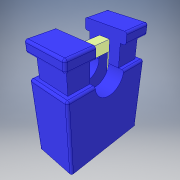
# Autodesk Inventor part: Jumper
Saved by Autodesk Inventor 2018 (Build 220112000, 112)
## iProperties
Created: 2021-02-06
Part Number: Jumper
Material: Všeobecné
Document SubType Name: Modeling
Designer: Jozko Mrkvicka
Density: 1 g/cm^3
Appearance: Výchozí
Author: Jozko Mrkvicka
Autodesk Inventor part; units mm, degrees
ref_plane "YZ Plane" through (0, 0, 0) normal (1, 0, 0) x (0, 1, 0)
ref_plane "XZ Plane" through (0, 0, 0) normal (0, 1, 0) x (-1, 0, 0)
ref_plane "XY Plane" through (0, 0, 0) normal (0, 0, 1) x (1, 0, 0)
sketch "Náčrt1" plane through (0, 0, 0) normal (0, 1, 0) x (-1, 0, 0)
  line L0 (0, 0) -> (2.54, 0)
  line L1 (2.54, 0) -> (2.54, -5.08)
  line L2 (2.54, -5.08) -> (0, -5.08)
  line L3 (0, -5.08) -> (0, 0)
  dimension "d0" = 2.54
  dimension "d1" = 5.08
  constraints: 8 end point, 2 parallel, 1 horizontal, 1 perpendicular
  measures "d0" distance of L1.end L2.end
  measures "d1" distance of L0.end L1.end
extrude "Vysunutí1" add sketch "Náčrt1" along normal blind 6.35
sketch "Náčrt2" plane through (0, 0, 0) normal (0, -1, 0) x (1, 0, 0)
  line L0 (-0.635, -0.635) -> (-1.905, -0.635)
  line L1 (-1.905, -0.635) -> (-1.905, -4.445)
  line L2 (-1.905, -4.445) -> (-0.635, -4.445)
  line L3 (-0.635, -4.445) -> (-0.635, -0.635)
  line L4 (-0.9525, -0.9525) -> (-1.5875, -0.9525)
  line L5 (-1.5875, -0.9525) -> (-1.5875, -4.1275)
  line L6 (-1.5875, -4.1275) -> (-0.9525, -4.1275)
  line L7 (-0.9525, -4.1275) -> (-0.9525, -0.9525)
  constraints: 16 end point, 4 parallel, 2 horizontal, 2 perpendicular
extrude "Vysunutí2" cut sketch "Náčrt2" against normal blind 0.635
sketch "Náčrt3" plane through (0, 0, 0) normal (1, 0, 0) x (0, 0, -1)
  line L0 (0, 6.35) -> (5.08, 6.35) projected
  line L1 (3.4925, 6.35) -> (3.4925, 4.445)
  line L2 (1.5875, 4.445) -> (1.5875, 6.35)
  arc A0 (1.5875, 4.445) -> (3.4925, 4.445) centre (2.54, 4.445) ccw
  line L3 (5.08, 6.35) -> (0, 6.35) projected
  line L4 (1.5875, 6.35) -> (3.4925, 6.35)
  point P0 (2.54, 6.35)
  dimension "d31" = 1.905
  dimension "d32" = 1.905
  dimension "d33" = 0.9525
  constraints: 6 end point, 2 point on circle, 2 point on line, 1 centre point, 1 midpoint, 1 parallel
  measures "d31" distance of L2.start L2.end
  measures "d32" distance of L1.start L1.end
  measures "d33" radius of A0
extrude "Vysunutí3" cut sketch "Náčrt3" against normal up to next
sketch "Náčrt4" plane through (0, 0, 0) normal (0, -1, 0) x (1, 0, 0)
  line L0 (-1.5875, -0.9525) -> (-1.5875, -4.1275) projected
  line L1 (-0.9525, -0.9525) -> (-1.5875, -0.9525)
  line L2 (-1.5875, -0.9525) -> (-1.5875, -4.1275)
  line L3 (-1.5875, -4.1275) -> (-0.9525, -4.1275)
  line L4 (-0.9525, -4.1275) -> (-0.9525, -0.9525)
  point P0 (0, 0)
  constraints: 8 end point, 2 parallel, 1 horizontal, 1 perpendicular
extrude "Vysunutí4" cut sketch "Náčrt4" against normal blind 5.715
sketch "Náčrt5" plane through (-2.54, 0, 0) normal (0, 0, 1) x (1, 0, 0)
  line L0 (2.54, 0) -> (2.54, 6.35) projected
  line L1 (0, 0) -> (0, 6.35) projected
  line L2 (2.54, 5.715) -> (2.54, 5.08)
  line L3 (0, 5.08) -> (0, 5.715)
  line L4 (0, 5.715) -> (0.3175, 5.715)
  line L5 (0.3175, 5.715) -> (0.3175, 4.445)
  line L6 (0.3175, 4.445) -> (0, 4.445)
  line L7 (0, 4.445) -> (0, 5.715)
  line L8 (2.54, 5.715) -> (2.2225, 5.715)
  line L9 (2.2225, 5.715) -> (2.2225, 4.445)
  line L10 (2.2225, 4.445) -> (2.54, 4.445)
  line L11 (2.54, 4.445) -> (2.54, 5.715)
  line L12 (0, 6.35) -> (2.54, 6.35) projected
  dimension "d20" = 0.3175
  dimension "d21" = 0.3175
  dimension "d34" = 1.27
  dimension "d35" = 0.635
  dimension "d36" = 0.635
  dimension "d37" = 1.27
  constraints: 20 end point, 5 parallel, 2 horizontal, 2 perpendicular, 2 point on line
  measures "d20" distance of L5.end L6.end
  measures "d21" distance of L10.end L9.end
  measures "d34" distance of L4.end L5.end
  measures "d35" distance between parallel lines of L12 L4
  measures "d36" distance between parallel lines of L12 L8
  measures "d37" distance of L8.end L9.end
extrude "Vysunutí5" cut sketch "Náčrt5" against normal up to surface (5.08 mm away)
sketch "Náčrt6" plane through (-2.2225, 4.445, -3.4925) normal (-1, 0, 0) x (0, 0, 1)
  line L0 (0, 0) -> (-1.5875, 0) projected
  line L1 (-1.5875, 1.27) -> (-1.27, 1.27)
  line L2 (-1.27, 1.27) -> (-1.27, 0)
  line L3 (-1.27, 0) -> (-1.5875, 0)
  line L4 (-1.5875, 0) -> (-1.5875, 1.27)
  line L5 (3.4925, 1.27) -> (3.4925, 0) projected
  line L6 (3.4925, 0) -> (-1.5875, 0) projected
  line L7 (3.4925, 1.27) -> (3.175, 1.27)
  line L8 (3.175, 1.27) -> (3.175, 0)
  line L9 (3.175, 0) -> (3.4925, 0)
  line L10 (3.4925, 0) -> (3.4925, 1.27)
  point P0 (3.4925, -4.445)
  point P1 (1.905, 0)
  dimension "d24" = 0.3175
  dimension "d25" = 0.3175
  constraints: 16 end point, 4 parallel, 2 horizontal, 2 perpendicular, 2 point on line
  measures "d24" distance of L2.end L3.end
  measures "d25" distance of L9.end L8.end
extrude "Vysunutí6" cut sketch "Náčrt6" against normal up to surface (1.905 mm away)
sketch "Náčrt7" plane through (-0.9525, 0.635, -0.9525) normal (0, 0, -1) x (-1, 0, 0)
  line L0 (0.635, 0) -> (0.635, 5.08) projected
  line L1 (0.635, 5.08) -> (0, 5.08) projected
  line L2 (0, 5.08) -> (0.635, 5.08)
  line L3 (0.635, 5.08) -> (0.635, 4.445)
  line L4 (0.635, 4.445) -> (0, 4.445)
  line L5 (0, 4.445) -> (0, 5.08)
  point P0 (-0.9525, -0.635)
  dimension "d28" = 0.635
  constraints: 8 end point, 2 parallel, 1 horizontal, 1 perpendicular, 1 point on line
  measures "d28" distance of L2.end L3.end
extrude "Vysunutí7" add sketch "Náčrt7" along normal up to next
fillet "Zaoblení1" radius 0.127 26 edges at (-2.54, 2.2225, -5.08) (0, 2.2225, -5.08) (-2.54, 2.2225, 0) (0, 2.2225, 0) (0, 6.0325, 0) (0, 6.0325, -5.08) (-2.54, 6.0325, 0) (-2.54, 6.0325, -5.08) (0, 4.445, -0.7938) (-1.27, 4.445, 0) (-2.54, 4.445, -0.7938) (-2.54, 4.445, -4.2863) (-1.27, 4.445, -5.08) (0, 4.445, -4.2863) (0, 5.715, -0.7938) (-1.27, 5.715, 0) (-2.54, 5.715, -0.7938) (-2.54, 5.715, -4.2862) (-1.27, 5.715, -5.08) (0, 5.715, -4.2862) (-2.54, 6.35, -4.2862) (-1.27, 6.35, -5.08) (0, 6.35, -4.2862) (0, 6.35, -0.7938) (-1.27, 6.35, 0) (-2.54, 6.35, -0.7937)
sketch "Náčrt8" plane through (0, 0.635, 0) normal (0, -1, 0) x (1, 0, 0)
  line L0 (-1.5875, -0.9525) -> (-1.5875, -4.1275) projected
  line L1 (-1.905, -0.635) -> (-0.635, -0.635) projected
  line L2 (-1.5875, -0.9525) -> (-0.9525, -0.9525)
  line L3 (-0.9525, -0.9525) -> (-0.9525, -0.635)
  line L4 (-0.9525, -0.635) -> (-1.5875, -0.635)
  line L5 (-1.5875, -0.635) -> (-1.5875, -0.9525)
  line L6 (-0.9525, -4.1275) -> (-0.9525, -0.9525) projected
  line L7 (-0.635, -4.445) -> (-1.905, -4.445) projected
  line L8 (-0.9525, -4.1275) -> (-1.5875, -4.1275)
  line L9 (-1.5875, -4.1275) -> (-1.5875, -4.445)
  line L10 (-1.5875, -4.445) -> (-0.9525, -4.445)
  line L11 (-0.9525, -4.445) -> (-0.9525, -4.1275)
  constraints: 16 end point, 4 parallel, 3 point on line, 2 horizontal, 2 perpendicular
extrude "Vysunutí8" add sketch "Náčrt8" along normal blind 0.254 contours L5 L1 L3 L2 | L8 L11 L7 L9
